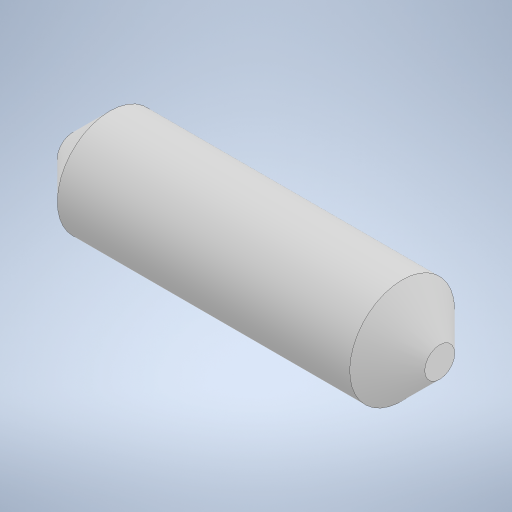
# Autodesk Inventor part: joint_3
Saved by Autodesk Inventor 2024 (Build 280153000, 153)
## iProperties
Created: 2024-03-11
Part Number: joint_3
Material: 일반
Document SubType Name: Modeling
Designer: SSAFY
Density: 1 g/cm^3
Appearance: 기본값
Author: SSAFY
Autodesk Inventor part; units mm, degrees
ref_plane "YZ Plane" through (0, 0, 0) normal (1, 0, 0) x (0, 1, 0)
ref_plane "XZ Plane" through (0, 0, 0) normal (0, 1, 0) x (-1, 0, 0)
ref_plane "XY Plane" through (0, 0, 0) normal (0, 0, 1) x (1, 0, 0)
sketch "스케치1" plane through (0, 0, 0) normal (0, 0, 1) x (1, 0, 0)
  line L0 (0, 0) -> (-9.8, 0)
  line L1 (-9.8, 0) -> (-9.8, 1.4)
  line L2 (-9.8, 1.4) -> (0, 1.4)
  line L3 (0, 1.4) -> (0, 0)
  dimension "d0" = 9.8
  dimension "d1" = 2.8
  constraints: 8 end point, 2 parallel, 1 horizontal, 1 perpendicular
  measures "d0" distance of L1.end L2.end
  measures "d1" diameter of L2 L0
revolve "회전1" add sketch "스케치1" angle 360 about axis through (0, 0, 0) along (-1, 0, 0)
chamfer "모따기1" distance 1 angle 45 2 edges at (0, -1.4, 0) (-9.8, -1.4, 0)
